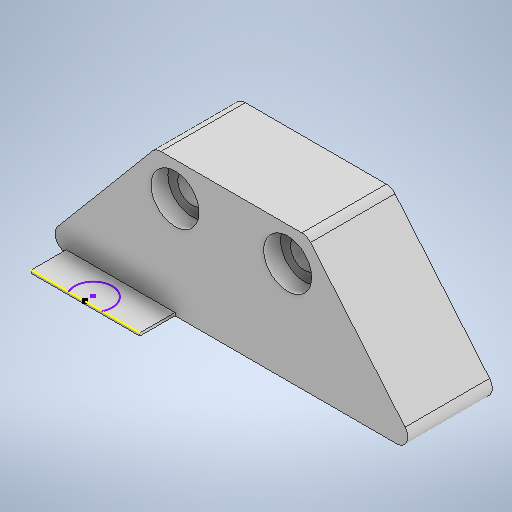
# Autodesk Inventor part: EngineMount
Saved by Autodesk Inventor 2026.1 (Build 301233020, 233B)
## iProperties
Created: 2025-10-14
Part Number: EngineMount
Material: Generic
Document SubType Name: Modeling
Designer: yo
Density: 1 g/cm^3
Appearance: Default
Author: yo
Autodesk Inventor part; units mm, degrees
ref_plane "YZ Plane" through (0, 0, 0) normal (1, 0, 0) x (0, 1, 0)
ref_plane "XZ Plane" through (0, 0, 0) normal (0, 1, 0) x (-1, 0, 0)
ref_plane "XY Plane" through (0, 0, 0) normal (0, 0, 1) x (1, 0, 0)
sketch "Sketch1" plane through (0, 0, 0) normal (0, 0, 1) x (1, 0, 0)
  line L0 (-58.5999, 0) -> (58.5999, 0)
  line L1 (-25.0359, 48) -> (25.0359, 48)
  circle A0 centre (-20, 36) radius 8.5
  line L2 (0, 48) -> (0, 0) construction
  circle A1 centre (-20, 36) radius 5
  circle A2 centre (20, 36) radius 8.5
  circle A3 centre (20, 36) radius 5
  arc A4 (-61.664, 6.5712) -> (-58.5999, 0) centre (-58.5999, 4) ccw
  arc A5 (-25.0359, 48) -> (-28.1, 46.5712) centre (-25.0359, 44) ccw
  line L3 (-61.664, 6.5712) -> (-28.1, 46.5712)
  arc A6 (58.5999, 0) -> (61.664, 6.5712) centre (58.5999, 4) ccw
  arc A7 (28.1, 46.5712) -> (25.0359, 48) centre (25.0359, 44) ccw
  line L4 (61.664, 6.5712) -> (28.1, 46.5712)
  line L5 (-58.5999, 1) -> (-19.9999, 1)
  line L6 (-19.9999, 1) -> (-19.9999, 0)
  line L7 (-19.9999, 0) -> (-58.5999, 0)
  line L8 (-58.5999, 0) -> (-58.5999, 1)
  point P0 (-58.5999, 0.5)
  point P1 (-39.2999, 0)
  point P2 (-19.9999, 0)
  dimension "d1" = 17
  dimension "d3" = 3.5
  dimension "d4" = 36
  dimension "d7" = 10
  dimension "d8" = 40
  dimension "d10" = 4
  dimension "d11" = 13
  dimension "d12" = 50
  dimension "d17" = 1
  dimension "d18" = 38.6
  constraints: 18 end point, 8 centre point, 8 point on circle, 6 symmetric about line, 4 coincident, 4 midpoint, 4 tangent, 3 horizontal, 2 parallel, 1 equal radius, 1 horizontal alignment, 1 perpendicular, 1 vertical, 1 vertical alignment, 4 other
  measures "d1" diameter of A0
  measures "d3" distance edge to line of A0 L1
  measures "d4" distance from line of L0 A0.centre
  measures "d7" diameter of A1
  measures "d8" distance of A2.centre A0.centre
  measures "d10" radius of A4
  measures "d11" distance from line of A0.centre L3
  measures "d12" angle of L0 L3
  measures "d17" distance of L5.end L6.end
  measures "d18" distance of L6.end L7.end
extrude "Extrusion1" add sketch "Sketch1" along normal mid plane 30 contours L8 L5 L6 L0 | A4 L3 A5 L1 A7 L4 A6 L0 L6 L5 L8
extrude "Extrusion2" add sketch "Sketch1" along normal mid plane 18 contours A0 | A2
extrude "Extrusion3" add sketch "Sketch1" along normal blind 27.5 contours L8 L5 L6 L0
sketch "Sketch2" plane through (-58.5999, 1, 15) normal (0, 1, 0) x (1, 0, 0)
  line L0 (0, -12.5) -> (38.6, -12.5) projected
  arc A0 (25.2908, -12.5) -> (13.3092, -12.5) centre (19.3, -9.6597) ccw
  point P0 (58.5999, 15)
  point P1 (19.3, -12.5)
  constraints: 2 point on circle, 2 point on line, 1 centre point, 1 midpoint, 1 vertical alignment
body "Solid1"
